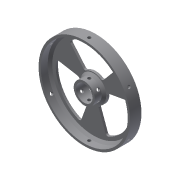
# Autodesk Inventor part: cellSTORM_Wheel_Micrometer
Saved by Autodesk Inventor 2019 (Build 230136000, 136)
## iProperties
Created: 2019-11-06
Part Number: cellSTORM_Wheel_Micrometer
Material: Generic
Document SubType Name: Modeling
Designer: diederichbenedict
Density: 1 g/cm^3
Appearance: Default
Author: diederichbenedict
Autodesk Inventor part; units mm, degrees
ref_plane "YZ Plane" through (0, 0, 0) normal (1, 0, 0) x (0, 1, 0)
ref_plane "XZ Plane" through (0, 0, 0) normal (0, 1, 0) x (-1, 0, 0)
ref_plane "XY Plane" through (0, 0, 0) normal (0, 0, 1) x (1, 0, 0)
sketch "Sketch1" plane through (0, 0, 0) normal (0, 0, 1) x (1, 0, 0)
  circle A0 centre (0, 0) radius 40
  circle A1 centre (0, 0) radius 7.25
  dimension "d0" = 80
  dimension "d1" = 14.5
  constraints: 2 centre point, 2 coincident
  measures "d0" diameter of A0
  measures "d1" diameter of A1
extrude "Extrusion1" add sketch "Sketch1" along normal blind 10
shell "Shell1" thickness 2 removed faces 1 at (-13.7905, -25.4111, 10)
chamfer "Chamfer1" distance 2 angle 45 2 edges at (-38, 0, 2) (-9.25, 0, 2)
sketch "Sketch2" plane through (0, 0, 0) normal (0, 1, 0) x (-1, 0, 0)
  line L0 (40, 10) -> (-40, 10) projected
  line L1 (-40, 0) -> (40, 0) projected
  circle A0 centre (0, 5.6678) radius 1.4
  point P0 (0, 0)
  dimension "d8" = 2.8
  constraints: 1 centre point
  measures "d8" diameter of A0
extrude "Extrusion2" cut sketch "Sketch2" along normal through all both and the other way through all
pattern_circular "Circular Pattern1" count 6 over 360 about axis through (0, 0, 0) along (0, 0, 1) of "Extrusion2"
sketch "Sketch3" plane through (0, 0, 2) normal (0, 0, 1) x (1, 0, 0)
  circle A0 centre (0, 0) radius 36 projected
  circle A1 centre (0, 0) radius 11.25 projected
  circle A2 centre (0, 0) radius 36 construction
  line L0 (0, 0) -> (23.1404, 27.5776) construction
  line L1 (0, 0) -> (36, 0) construction
  line L2 (23.1404, 27.5776) -> (0, 0) construction
  line L3 (-8.9067, 10.6146) -> (-19.8849, 23.6979) construction
  line L4 (0, 0) -> (17.079, 0) construction
  arc A3 (19.5369, 26.5953) -> (-19.5369, 26.5953) centre (0, 0) ccw
  arc A4 (6.3211, 10.2002) -> (-6.3211, 10.2002) centre (0, 0) ccw
  line L5 (-8.9067, 10.6146) -> (-19.8849, 23.6979)
  line L6 (8.9067, 10.6146) -> (19.8849, 23.6979)
  arc A5 (-19.5369, 26.5953) -> (-19.8849, 23.6979) centre (-18.3528, 24.9835) ccw
  arc A6 (-8.9067, 10.6146) -> (-6.3211, 10.2002) centre (-7.3746, 11.9002) ccw
  arc A7 (6.3211, 10.2002) -> (8.9067, 10.6146) centre (7.3746, 11.9002) ccw
  arc A8 (19.8849, 23.6979) -> (19.5369, 26.5953) centre (18.3528, 24.9835) ccw
  point P0 (21.212, 25.2795)
  point P1 (7.7135, 9.1925)
  dimension "d14" = 50
  dimension "d15" = 130
  dimension "d16" = 2
  dimension "d17" = 33
  dimension "d18" = 12
  constraints: 14 end point, 14 point on circle, 8 tangent, 6 centre point, 4 point on line, 3 collinear, 3 equal radius, 2 equal length, 2 horizontal, 1 coincident, 2 other
  measures "d14" angle of L1 L0
  measures "d15" angle of L4 L3
  measures "d16" radius of A5
  measures "d17" radius of A3
  measures "d18" radius of A4
extrude "Extrusion3" cut sketch "Sketch3" against normal blind 10 contours A8 L6 A7 A4 A6 L5 A5 A3
pattern_circular "Circular Pattern2" count 3 over 360 about axis through (0, 0, 0) along (0, 0, 1) of "Extrusion3"
body "Solid1"
